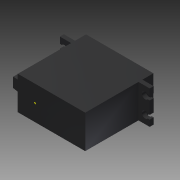
# Autodesk Inventor part: servo 13kg BMS-630MG
Saved by Autodesk Inventor 2013 (Build 170138000, 138)
## iProperties
Created: 2013-03-06
Part Number: servo 13kg BMS-630MG
Material: Generic
Document SubType Name: Modeling
Designer: Masta
Density: 1.52304 g/cm^3
Mass: 52 g
Surface Area: 75.1113 cm^2
Volume: 34.1422 cm^3
Author: Masta
Autodesk Inventor part; units mm, degrees
ref_plane "YZ Plane" through (0, 0, 0) normal (1, 0, 0) x (0, 1, 0)
ref_plane "XZ Plane" through (0, 0, 0) normal (0, 1, 0) x (-1, 0, 0)
ref_plane "XY Plane" through (0, 0, 0) normal (0, 0, 1) x (1, 0, 0)
sketch "Sketch1" plane through (0, 0, 0) normal (0, 1, 0) x (-1, 0, 0)
  line L0 (20.25, 10) -> (-20.25, 10)
  line L1 (-20.25, 10) -> (-20.25, -10)
  line L2 (-20.25, -10) -> (20.25, -10)
  line L3 (20.25, -10) -> (20.25, 10)
  line L4 (20.25, 10) -> (-20.25, -10) construction
  line L5 (-20.25, 10) -> (20.25, -10) construction
  line L6 (-27, 10) -> (-27, 6.25)
  line L7 (27, -10) -> (27, -6.25)
  line L8 (27, 10) -> (-27, -10) construction
  line L9 (-27, 10) -> (27, -10) construction
  line L10 (20.25, -10) -> (27, -10)
  line L11 (20.25, 10) -> (27, 10)
  line L12 (-20.25, 10) -> (-27, 10)
  line L13 (-20.25, -10) -> (-27, -10)
  line L14 (24.25, 5) -> (-24.25, 5) construction
  line L15 (-24.25, 5) -> (-24.25, -5) construction
  line L16 (-24.25, -5) -> (24.25, -5) construction
  line L17 (24.25, -5) -> (24.25, 5) construction
  line L18 (24.25, 5) -> (-24.25, -5) construction
  line L19 (-24.25, 5) -> (24.25, -5) construction
  circle A0 centre (-24.25, 5) radius 2
  line L20 (-27, 3.75) -> (-25.8112, 3.75)
  line L21 (-27, 6.25) -> (-25.8112, 6.25)
  line L22 (-20.25, 0) -> (20.25, 0) construction
  line L23 (0, 10) -> (0, -10) construction
  circle A1 centre (-24.25, -5) radius 2
  line L24 (-27, -3.75) -> (-25.8112, -3.75)
  line L25 (-27, -6.25) -> (-25.8112, -6.25)
  circle A2 centre (24.25, 5) radius 2
  line L26 (27, 3.75) -> (25.8112, 3.75)
  line L27 (27, 6.25) -> (25.8112, 6.25)
  line L28 (27, -6.25) -> (25.8112, -6.25)
  line L29 (27, -3.75) -> (25.8112, -3.75)
  circle A3 centre (24.25, -5) radius 2
  line L30 (-27, 3.75) -> (-27, -3.75)
  line L31 (-27, 6.25) -> (-27, 3.75)
  line L32 (-27, -6.25) -> (-27, -10)
  line L33 (-27, -3.75) -> (-27, -6.25)
  line L34 (27, -3.75) -> (27, 3.75)
  line L35 (27, -6.25) -> (27, -3.75)
  line L36 (27, 3.75) -> (27, 6.25)
  line L37 (27, 6.25) -> (27, 10)
  point P0 (0, 0)
  dimension "d0" = 40.5
  dimension "d1" = 20
  dimension "d2" = 54
  dimension "d3" = 48.5
  dimension "d4" = 10
  dimension "d12" = 2.5
  dimension "d13" = 4
  constraints: 76 end point, 32 parallel, 15 symmetric about line, 12 perpendicular, 10 midpoint, 8 point on circle, 4 centre point, 2 collinear, 2 horizontal, 1 coincident, 4 other
  measures "d0" distance of L2.end L1.end
  measures "d1" distance of L1.end L0.end
  measures "d2" distance of L7.start L8.end
  measures "d3" distance of L16.end L15.end
  measures "d4" distance of L15.end L14.end
  measures "d12" distance between parallel lines of L20 L21
  measures "d13" diameter of A0
extrude "Extrusion1" add sketch "Sketch1" along normal blind 9 and the other way blind 32 contours L3 L2 L1 L0
extrude "Extrusion2" add sketch "Sketch1" along normal blind 2.4 contours L11 L37 L27 A2 L26 L34 L29 A3 L28 L7 L10 L3 | L1 L13 L32 L25 A1 L24 L30 L20 A0 L21 L6 L12
sketch "Sketch2" plane through (0, 9, 0) normal (0, 1, 0) x (1, 0, 0)
  line L0 (-20.25, 10) -> (-20.25, -10) projected
  circle A0 centre (-9.75, 0) radius 6
  line L1 (-9.75, 0) -> (0, 0) construction
  dimension "d14" = 12
  dimension "d15" = 10.5
  constraints: 2 end point, 1 centre point, 1 perpendicular
  measures "d14" diameter of A0
  measures "d15" distance from line of L1.start L0
extrude "Extrusion3" add sketch "Sketch2" along normal blind 1.5
sketch "Sketch3" plane through (-9.75, 10.5, 0) normal (0, 1, 0) x (1, 0, 0)
  circle A0 centre (0, 0) radius 6 projected
  circle A1 centre (0, 0) radius 3
  point P0 (9.75, 0)
  dimension "d18" = 6
  constraints: 1 centre point, 1 coincident
  measures "d18" diameter of A1
extrude "Extrusion4" add sketch "Sketch3" along normal blind 4 contours A1
sketch "Sketch4" plane through (-20.25, -32, -10) normal (-1, 0, 0) x (0, 0, 1)
  line L0 (20, 32) -> (0, 32) projected
  line L1 (6.5, 3.5) -> (13.5, 3.5)
  line L2 (13.5, 3.5) -> (13.5, 8)
  line L3 (13.5, 8) -> (6.5, 8)
  line L4 (6.5, 8) -> (6.5, 3.5)
  line L5 (6.5, 3.5) -> (13.5, 8) construction
  line L6 (13.5, 3.5) -> (6.5, 8) construction
  line L7 (10, 32) -> (10, 5.75) construction
  dimension "d21" = 7
  dimension "d22" = 4.5
  dimension "d23" = 24
  constraints: 14 end point, 3 parallel, 2 midpoint, 1 horizontal, 1 perpendicular
  measures "d21" distance of L3.end L2.end
  measures "d22" distance of L2.end L1.end
  measures "d23" distance between parallel lines of L0 L3
extrude "Extrusion5" add sketch "Sketch4" along normal blind 7 draft -5
sketch "Sketch5" plane through (0, 0, 0) normal (0, 0, 1) x (1, 0, 0)
  line L0 (27, 2.4) -> (27, 0) projected
  line L1 (27, 0) -> (20.25, 0) projected
  line L2 (20.25, 0) -> (20.25, -32) projected
  line L3 (20.25, -32) -> (-20.25, -32) projected
  line L4 (-20.25, -32) -> (-20.25, -28.5) projected
  line L5 (-20.25, -28.5) -> (-27.25, -27.8876) projected
  line L6 (-27.25, -27.8876) -> (-27.25, -24.6124) projected
  line L7 (-27.25, -24.6124) -> (-20.25, -24) projected
  line L8 (-20.25, -24) -> (-20.25, 0) projected
  line L9 (-20.25, 0) -> (-27, 0) projected
  line L10 (-27, 0) -> (-27, 2.4) projected
  line L11 (-27, 2.4) -> (-20.25, 2.4) projected
  line L12 (-20.25, 2.4) -> (-20.25, 9) projected
  line L13 (-20.25, 9) -> (-15.75, 9) projected
  line L14 (-15.75, 9) -> (-15.75, 10.5) projected
  line L15 (-15.75, 10.5) -> (-12.75, 10.5) projected
  line L16 (-12.75, 10.5) -> (-12.75, 14.5) projected
  line L17 (-12.75, 14.5) -> (-6.75, 14.5) projected
  line L18 (-6.75, 14.5) -> (-6.75, 10.5) projected
  line L19 (-6.75, 10.5) -> (-3.75, 10.5) projected
  line L20 (-3.75, 10.5) -> (-3.75, 9) projected
  line L21 (-3.75, 9) -> (20.25, 9) projected
  line L22 (20.25, 9) -> (20.25, 2.4) projected
  line L23 (20.25, 2.4) -> (27, 2.4) projected
  line L24 (-27, 2.4) -> (-20.25, 3.5)
  line L25 (20.25, 3.5) -> (27, 2.4)
  point P0 (0, 0)
  dimension "d26" = 1.1
  constraints: 4 end point, 2 point on line, 1 equal length
  measures "d26" distance of L24.end L11.end
extrude "Extrusion6" add sketch "Sketch5" along normal mid plane 1.3 contours L23 L22 L25 | L24 L12 L11
sketch "Sketch6" plane through (0, 9, 0) normal (0, 1, 0) x (1, 0, 0)
  line L0 (12.3297, -9.4801) -> (12.3297, 4.6475) construction
  line L1 (12.3297, 4.6475) -> (15.9034, 4.6475) construction
  line L2 (15.9034, 4.6475) -> (15.9034, -9.4801) construction
  line L3 (15.9034, -9.4801) -> (12.3297, -9.4801) construction
  spline S0 degree 2 poles (14.1431, -7.5) (14.3325, -7.5) (14.6227, -7.6441) (14.7174, -7.7634) knots 0 0 0 1 2 2 2
  spline S1 degree 2 poles (14.7174, -7.7634) (14.8285, -7.9075) (14.9232, -8.2348) (14.9232, -8.4942) knots 0 0 0 1 2 2 2
  line L4 (14.9232, -8.4942) -> (14.9232, -9.2228)
  line L5 (14.9232, -9.2228) -> (12.3832, -9.2228)
  line L6 (12.3832, -9.2228) -> (12.3832, -8.5497)
  spline S2 degree 2 poles (12.3832, -8.5497) (12.3832, -8.278) (12.4182, -8.0063) (12.4861, -7.8828) knots 0 0 0 1 2 2 2
  spline S3 degree 2 poles (12.4861, -7.8828) (12.5582, -7.7449) (12.7949, -7.6194) (12.9554, -7.6194) knots 0 0 0 1 2 2 2
  spline S4 degree 2 poles (12.9554, -7.6194) (13.1345, -7.6194) (13.4185, -7.8087) (13.4988, -7.9755) knots 0 0 0 1 2 2 2
  line L7 (13.4988, -7.9755) -> (13.5112, -7.9755)
  spline S5 degree 2 poles (13.5112, -7.9755) (13.5729, -7.749) (13.9002, -7.5) (14.1431, -7.5) knots 0 0 0 1 2 2 2
  spline S6 degree 2 poles (14.1575, -7.852) (14.0134, -7.852) (13.8282, -7.9343) (13.7623, -8.0578) knots 0 0 0 1 2 2 2
  spline S7 degree 2 poles (13.7623, -8.0578) (13.7211, -8.1381) (13.6964, -8.3274) (13.6964, -8.5024) knots 0 0 0 1 2 2 2
  line L8 (13.6964, -8.5024) -> (13.6964, -8.8852)
  line L9 (13.6964, -8.8852) -> (14.635, -8.8852)
  line L10 (14.635, -8.8852) -> (14.635, -8.6115)
  spline S8 degree 2 poles (14.635, -8.6115) (14.635, -8.3892) (14.5939, -8.1339) (14.528, -8.0351) knots 0 0 0 1 2 2 2
  spline S9 degree 2 poles (14.528, -8.0351) (14.4601, -7.9405) (14.2913, -7.852) (14.1575, -7.852) knots 0 0 0 1 2 2 2
  spline S10 degree 2 poles (13.0028, -7.9713) (12.9122, -7.9713) (12.7763, -8.0331) (12.7372, -8.101) knots 0 0 0 1 2 2 2
  spline S11 degree 2 poles (12.7372, -8.101) (12.692, -8.1833) (12.6714, -8.383) (12.6714, -8.5621) knots 0 0 0 1 2 2 2
  line L11 (12.6714, -8.5621) -> (12.6714, -8.8852)
  line L12 (12.6714, -8.8852) -> (13.4144, -8.8852)
  line L13 (13.4144, -8.8852) -> (13.4144, -8.5024)
  spline S12 degree 2 poles (13.4144, -8.5024) (13.4144, -8.3439) (13.3815, -8.1936) (13.33, -8.1134) knots 0 0 0 1 2 2 2
  spline S13 degree 2 poles (13.33, -8.1134) (13.2806, -8.0351) (13.1221, -7.9713) (13.0028, -7.9713) knots 0 0 0 1 2 2 2
  line L14 (14.9232, -4.9867) -> (14.9232, -5.3243)
  line L15 (14.9232, -5.3243) -> (12.7352, -5.3243)
  line L16 (12.7352, -5.3243) -> (14.2234, -5.9871)
  line L17 (14.2234, -5.9871) -> (14.2234, -6.1929)
  line L18 (14.2234, -6.1929) -> (12.7352, -6.8495)
  line L19 (12.7352, -6.8495) -> (14.9232, -6.8495)
  line L20 (14.9232, -6.8495) -> (14.9232, -7.1645)
  line L21 (14.9232, -7.1645) -> (12.3832, -7.1645)
  line L22 (12.3832, -7.1645) -> (12.3832, -6.7034)
  line L23 (12.3832, -6.7034) -> (13.7973, -6.0694)
  line L24 (13.7973, -6.0694) -> (12.3832, -5.456)
  line L25 (12.3832, -5.456) -> (12.3832, -4.9867)
  line L26 (12.3832, -4.9867) -> (14.9232, -4.9867)
  spline S14 degree 2 poles (14.9685, -3.7641) (14.9685, -4.0399) (14.8532, -4.4269) (14.7709, -4.5977) knots 0 0 0 1 2 2 2
  line L27 (14.7709, -4.5977) -> (14.3469, -4.5977)
  line L28 (14.3469, -4.5977) -> (14.3469, -4.573)
  spline S15 degree 2 poles (14.3469, -4.573) (14.5033, -4.4063) (14.6762, -3.9843) (14.6762, -3.7888) knots 0 0 0 1 2 2 2
  spline S16 degree 2 poles (14.6762, -3.7888) (14.6762, -3.5088) (14.4436, -3.2227) (14.2522, -3.2227) knots 0 0 0 1 2 2 2
  spline S17 degree 2 poles (14.2522, -3.2227) (14.0999, -3.2227) (13.9105, -3.373) (13.8632, -3.5356) knots 0 0 0 1 2 2 2
  spline S18 degree 2 poles (13.8632, -3.5356) (13.8302, -3.6529) (13.7849, -3.8485) (13.7479, -3.9946) knots 0 0 0 1 2 2 2
  spline S19 degree 2 poles (13.7479, -3.9946) (13.7129, -4.1263) (13.6079, -4.3342) (13.5235, -4.4145) knots 0 0 0 1 2 2 2
  spline S20 degree 2 poles (13.5235, -4.4145) (13.4391, -4.4927) (13.2127, -4.5792) (13.0645, -4.5792) knots 0 0 0 1 2 2 2
  spline S21 degree 2 poles (13.0645, -4.5792) (12.7558, -4.5792) (12.3379, -4.0975) (12.3379, -3.725) knots 0 0 0 1 2 2 2
  spline S22 degree 2 poles (12.3379, -3.725) (12.3379, -3.5109) (12.4223, -3.1322) (12.5026, -2.9696) knots 0 0 0 1 2 2 2
  line L29 (12.5026, -2.9696) -> (12.906, -2.9696)
  line L30 (12.906, -2.9696) -> (12.906, -2.9943)
  spline S23 degree 2 poles (12.906, -2.9943) (12.7949, -3.1157) (12.6302, -3.4944) (12.6302, -3.7023) knots 0 0 0 1 2 2 2
  spline S24 degree 2 poles (12.6302, -3.7023) (12.6302, -3.937) (12.8504, -4.2272) (13.0295, -4.2272) knots 0 0 0 1 2 2 2
  spline S25 degree 2 poles (13.0295, -4.2272) (13.1901, -4.2272) (13.3815, -4.0564) (13.4247, -3.8958) knots 0 0 0 1 2 2 2
  spline S26 degree 2 poles (13.4247, -3.8958) (13.4535, -3.7888) (13.5276, -3.478) (13.5585, -3.375) knots 0 0 0 1 2 2 2
  spline S27 degree 2 poles (13.5585, -3.375) (13.6388, -3.1136) (13.962, -2.8708) (14.1987, -2.8708) knots 0 0 0 1 2 2 2
  spline S28 degree 2 poles (14.1987, -2.8708) (14.3489, -2.8708) (14.6371, -2.9922) (14.7379, -3.1013) knots 0 0 0 1 2 2 2
  spline S29 degree 2 poles (14.7379, -3.1013) (14.8491, -3.2227) (14.9685, -3.5315) (14.9685, -3.7641) knots 0 0 0 1 2 2 2
  line L31 (13.9661, -1.6687) -> (13.9661, -2.6299)
  line L32 (13.9661, -2.6299) -> (13.6573, -2.6299)
  line L33 (13.6573, -2.6299) -> (13.6573, -1.6687)
  line L34 (13.6573, -1.6687) -> (13.9661, -1.6687)
  spline S30 degree 2 poles (14.0999, 0.2744) (14.2954, 0.2744) (14.6268, 0.1447) (14.7379, 0.0356) knots 0 0 0 1 2 2 2
  spline S31 degree 2 poles (14.7379, 0.0356) (14.8553, -0.0776) (14.9767, -0.3616) (14.9767, -0.5325) knots 0 0 0 1 2 2 2
  spline S32 degree 2 poles (14.9767, -0.5325) (14.9767, -0.7033) (14.8614, -0.9853) (14.7462, -1.0923) knots 0 0 0 1 2 2 2
  spline S33 degree 2 poles (14.7462, -1.0923) (14.6083, -1.2241) (14.1451, -1.3723) (13.8076, -1.3723) knots 0 0 0 1 2 2 2
  spline S34 degree 2 poles (13.8076, -1.3723) (13.4762, -1.3723) (12.9431, -1.2364) (12.7455, -1.0944) knots 0 0 0 1 2 2 2
  spline S35 degree 2 poles (12.7455, -1.0944) (12.552, -0.9565) (12.3359, -0.5201) (12.3359, -0.234) knots 0 0 0 1 2 2 2
  spline S36 degree 2 poles (12.3359, -0.234) (12.3359, -0.1496) (12.3523, -0.0014) (12.3708, 0.0542) knots 0 0 0 1 2 2 2
  line L35 (12.3708, 0.0542) -> (12.6981, 0.0542)
  line L36 (12.6981, 0.0542) -> (12.6981, 0.0397)
  spline S37 degree 2 poles (12.6981, 0.0397) (12.6734, -0.0076) (12.6302, -0.1805) (12.6302, -0.2793) knots 0 0 0 1 2 2 2
  spline S38 degree 2 poles (12.6302, -0.2793) (12.6302, -0.5963) (13.0583, -0.9853) (13.4782, -1.0224) knots 0 0 0 1 2 2 2
  spline S39 degree 2 poles (13.4782, -1.0224) (13.3938, -0.9009) (13.3012, -0.6457) (13.3012, -0.4934) knots 0 0 0 1 2 2 2
  spline S40 degree 2 poles (13.3012, -0.4934) (13.3012, -0.3452) (13.3609, -0.1229) (13.4515, -0.0014) knots 0 0 0 1 2 2 2
  spline S41 degree 2 poles (13.4515, -0.0014) (13.5565, 0.1385) (13.8817, 0.2744) (14.0999, 0.2744) knots 0 0 0 1 2 2 2
  spline S42 degree 2 poles (14.1143, -0.0714) (13.9578, -0.0714) (13.7458, -0.1537) (13.6717, -0.2443) knots 0 0 0 1 2 2 2
  spline S43 degree 2 poles (13.6717, -0.2443) (13.6182, -0.3122) (13.5832, -0.481) (13.5832, -0.5695) knots 0 0 0 1 2 2 2
  spline S44 degree 2 poles (13.5832, -0.5695) (13.5832, -0.6889) (13.6553, -0.9133) (13.7232, -1.0224) knots 0 0 0 1 2 2 2
  spline S45 degree 2 poles (13.7232, -1.0224) (13.7602, -1.0244) (13.8302, -1.0285) (13.8837, -1.0285) knots 0 0 0 1 2 2 2
  spline S46 degree 2 poles (13.8837, -1.0285) (14.1472, -1.0285) (14.4704, -0.9256) (14.5548, -0.8474) knots 0 0 0 1 2 2 2
  spline S47 degree 2 poles (14.5548, -0.8474) (14.635, -0.7754) (14.6988, -0.6189) (14.6988, -0.5304) knots 0 0 0 1 2 2 2
  spline S48 degree 2 poles (14.6988, -0.5304) (14.6988, -0.3246) (14.4066, -0.0714) (14.1143, -0.0714) knots 0 0 0 1 2 2 2
  spline S49 degree 2 poles (12.624, 1.2603) (12.624, 1.1677) (12.6693, 0.9845) (12.7043, 0.896) knots 0 0 0 1 2 2 2
  spline S50 degree 2 poles (12.7043, 0.896) (12.7393, 0.8137) (12.8134, 0.6922) (12.8463, 0.6449) knots 0 0 0 1 2 2 2
  line L37 (12.8463, 0.6449) -> (12.8463, 0.6243)
  line L38 (12.8463, 0.6243) -> (12.4861, 0.6243)
  spline S51 degree 2 poles (12.4861, 0.6243) (12.4264, 0.7355) (12.3297, 1.1163) (12.3297, 1.2871) knots 0 0 0 1 2 2 2
  spline S52 degree 2 poles (12.3297, 1.2871) (12.3297, 1.46) (12.3997, 1.7173) (12.4738, 1.8223) knots 0 0 0 1 2 2 2
  spline S53 degree 2 poles (12.4738, 1.8223) (12.554, 1.9334) (12.7866, 2.0487) (12.9431, 2.0487) knots 0 0 0 1 2 2 2
  spline S54 degree 2 poles (12.9431, 2.0487) (13.153, 2.0487) (13.47, 1.7729) (13.5112, 1.5794) knots 0 0 0 1 2 2 2
  line L39 (13.5112, 1.5794) -> (13.5359, 1.5794)
  spline S55 degree 2 poles (13.5359, 1.5794) (13.5523, 1.6597) (13.6264, 1.8429) (13.7005, 1.9211) knots 0 0 0 1 2 2 2
  spline S56 degree 2 poles (13.7005, 1.9211) (13.7726, 1.9993) (14.0031, 2.0981) (14.1698, 2.0981) knots 0 0 0 1 2 2 2
  spline S57 degree 2 poles (14.1698, 2.0981) (14.3407, 2.0981) (14.6309, 1.9808) (14.7421, 1.8737) knots 0 0 0 1 2 2 2
  spline S58 degree 2 poles (14.7421, 1.8737) (14.8573, 1.7626) (14.9767, 1.4477) (14.9767, 1.248) knots 0 0 0 1 2 2 2
  spline S59 degree 2 poles (14.9767, 1.248) (14.9767, 1.0566) (14.8841, 0.682) (14.8203, 0.5543) knots 0 0 0 1 2 2 2
  line L40 (14.8203, 0.5543) -> (14.4601, 0.5543)
  line L41 (14.4601, 0.5543) -> (14.4601, 0.579)
  spline S60 degree 2 poles (14.4601, 0.579) (14.5383, 0.6861) (14.6824, 1.0483) (14.6824, 1.2274) knots 0 0 0 1 2 2 2
  spline S61 degree 2 poles (14.6824, 1.2274) (14.6824, 1.3324) (14.6165, 1.5423) (14.5403, 1.6123) knots 0 0 0 1 2 2 2
  spline S62 degree 2 poles (14.5403, 1.6123) (14.4642, 1.6803) (14.2831, 1.7523) (14.1451, 1.7523) knots 0 0 0 1 2 2 2
  spline S63 degree 2 poles (14.1451, 1.7523) (14.0072, 1.7523) (13.8282, 1.672) (13.7767, 1.6) knots 0 0 0 1 2 2 2
  spline S64 degree 2 poles (13.7767, 1.6) (13.7252, 1.5279) (13.6861, 1.3324) (13.6861, 1.2171) knots 0 0 0 1 2 2 2
  line L42 (13.6861, 1.2171) -> (13.6861, 1.073)
  line L43 (13.6861, 1.073) -> (13.4041, 1.073)
  line L44 (13.4041, 1.073) -> (13.4041, 1.1862)
  spline S65 degree 2 poles (13.4041, 1.1862) (13.4041, 1.4147) (13.186, 1.7029) (12.9781, 1.7029) knots 0 0 0 1 2 2 2
  spline S66 degree 2 poles (12.9781, 1.7029) (12.8813, 1.7029) (12.7434, 1.6288) (12.7022, 1.5691) knots 0 0 0 1 2 2 2
  spline S67 degree 2 poles (12.7022, 1.5691) (12.659, 1.5053) (12.624, 1.3489) (12.624, 1.2603) knots 0 0 0 1 2 2 2
  spline S68 degree 2 poles (13.6532, 4.0618) (14.3366, 4.0618) (14.9767, 3.6645) (14.9767, 3.2508) knots 0 0 0 1 2 2 2
  spline S69 degree 2 poles (14.9767, 3.2508) (14.9767, 2.8309) (14.3242, 2.4377) (13.6553, 2.4377) knots 0 0 0 1 2 2 2
  spline S70 degree 2 poles (13.6553, 2.4377) (12.9678, 2.4377) (12.3317, 2.835) (12.3317, 3.2508) knots 0 0 0 1 2 2 2
  spline S71 degree 2 poles (12.3317, 3.2508) (12.3317, 3.6686) (12.9904, 4.0618) (13.6532, 4.0618) knots 0 0 0 1 2 2 2
  spline S72 degree 2 poles (14.4271, 3.6254) (14.3016, 3.6748) (13.9146, 3.716) (13.6532, 3.716) knots 0 0 0 1 2 2 2
  spline S73 degree 2 poles (13.6532, 3.716) (13.3918, 3.716) (13.0069, 3.6748) (12.8772, 3.6233) knots 0 0 0 1 2 2 2
  spline S74 degree 2 poles (12.8772, 3.6233) (12.7475, 3.5719) (12.6137, 3.3928) (12.6137, 3.2508) knots 0 0 0 1 2 2 2
  spline S75 degree 2 poles (12.6137, 3.2508) (12.6137, 3.1087) (12.7475, 2.9256) (12.8813, 2.872) knots 0 0 0 1 2 2 2
  spline S76 degree 2 poles (12.8813, 2.872) (13.011, 2.8206) (13.4062, 2.7835) (13.6553, 2.7835) knots 0 0 0 1 2 2 2
  spline S77 degree 2 poles (13.6553, 2.7835) (13.9228, 2.7835) (14.281, 2.8165) (14.421, 2.87) knots 0 0 0 1 2 2 2
  spline S78 degree 2 poles (14.421, 2.87) (14.5527, 2.9194) (14.6947, 3.1026) (14.6947, 3.2508) knots 0 0 0 1 2 2 2
  spline S79 degree 2 poles (14.6947, 3.2508) (14.6947, 3.3907) (14.5609, 3.5739) (14.4271, 3.6254) knots 0 0 0 1 2 2 2
  line L45 (14.9232, 6.6368) -> (14.9232, 6.2992)
  line L46 (14.9232, 6.2992) -> (12.7352, 6.2992)
  line L47 (12.7352, 6.2992) -> (14.2234, 5.6364)
  line L48 (14.2234, 5.6364) -> (14.2234, 5.4306)
  line L49 (14.2234, 5.4306) -> (12.7352, 4.7739)
  line L50 (12.7352, 4.7739) -> (14.9232, 4.7739)
  line L51 (14.9232, 4.7739) -> (14.9232, 4.459)
  line L52 (14.9232, 4.459) -> (12.3832, 4.459)
  line L53 (12.3832, 4.459) -> (12.3832, 4.9201)
  line L54 (12.3832, 4.9201) -> (13.7973, 5.5541)
  line L55 (13.7973, 5.5541) -> (12.3832, 6.1674)
  line L56 (12.3832, 6.1674) -> (12.3832, 6.6368)
  line L57 (12.3832, 6.6368) -> (14.9232, 6.6368)
  spline S80 degree 2 poles (14.9726, 8.2155) (14.9726, 7.9459) (14.8079, 7.4992) (14.6412, 7.3386) knots 0 0 0 1 2 2 2
  spline S81 degree 2 poles (14.6412, 7.3386) (14.4724, 7.1781) (13.9743, 7.0073) (13.6511, 7.0073) knots 0 0 0 1 2 2 2
  spline S82 degree 2 poles (13.6511, 7.0073) (13.3444, 7.0073) (12.8587, 7.1802) (12.6858, 7.3407) knots 0 0 0 1 2 2 2
  spline S83 degree 2 poles (12.6858, 7.3407) (12.5191, 7.4951) (12.3379, 7.9479) (12.3379, 8.2176) knots 0 0 0 1 2 2 2
  spline S84 degree 2 poles (12.3379, 8.2176) (12.3379, 8.3472) (12.375, 8.5819) (12.4079, 8.6889) knots 0 0 0 1 2 2 2
  spline S85 degree 2 poles (12.4079, 8.6889) (12.4326, 8.7754) (12.5232, 8.9853) (12.5561, 9.0491) knots 0 0 0 1 2 2 2
  line L58 (12.5561, 9.0491) -> (12.9637, 9.0491)
  line L59 (12.9637, 9.0491) -> (12.9637, 9.0203)
  spline S86 degree 2 poles (12.9637, 9.0203) (12.9081, 8.9565) (12.8072, 8.8227) (12.7496, 8.6992) knots 0 0 0 1 2 2 2
  spline S87 degree 2 poles (12.7496, 8.6992) (12.6981, 8.5963) (12.6302, 8.3308) (12.6302, 8.1785) knots 0 0 0 1 2 2 2
  spline S88 degree 2 poles (12.6302, 8.1785) (12.6302, 7.8121) (13.1818, 7.3592) (13.6408, 7.3592) knots 0 0 0 1 2 2 2
  spline S89 degree 2 poles (13.6408, 7.3592) (13.8961, 7.3592) (14.2789, 7.4786) (14.4107, 7.5918) knots 0 0 0 1 2 2 2
  spline S90 degree 2 poles (14.4107, 7.5918) (14.5424, 7.7009) (14.6803, 8.0097) (14.6803, 8.2032) knots 0 0 0 1 2 2 2
  spline S91 degree 2 poles (14.6803, 8.2032) (14.6803, 8.3452) (14.6391, 8.6292) (14.598, 8.726) knots 0 0 0 1 2 2 2
  line L60 (14.598, 8.726) -> (13.9414, 8.726)
  line L61 (13.9414, 8.726) -> (13.9414, 8.1373)
  line L62 (13.9414, 8.1373) -> (13.645, 8.1373)
  line L63 (13.645, 8.1373) -> (13.645, 9.0594)
  line L64 (13.645, 9.0594) -> (14.7544, 9.0594)
  spline S92 degree 2 poles (14.7544, 9.0594) (14.7832, 8.9956) (14.8717, 8.7774) (14.8985, 8.6848) knots 0 0 0 1 2 2 2
  spline S93 degree 2 poles (14.8985, 8.6848) (14.9355, 8.5592) (14.9726, 8.3575) (14.9726, 8.2155) knots 0 0 0 1 2 2 2
  point P0 (0, 0)
  constraints: 2 other
emboss "Emboss1" sketch "Sketch6" operation cut depth 0.1 direction (0, -1, 0)
hole "Hole1" at (-9.75, 14.5, 0) direction (0, -1, 0) diameter 2.459 depth 8 tip angle 118 thread size "M3x0.5" class "6H" standard "ISO Metric profile"
sketch "Sketch7" plane through (0, -32, 0) normal (0, -1, 0) x (1, 0, 0)
  line L0 (20.25, 10) -> (-20.25, 10) projected
  line L1 (-20.25, 10) -> (-20.25, -10) projected
  line L2 (-20.25, -10) -> (20.25, -10) projected
  line L3 (20.25, -10) -> (20.25, 10) projected
  point P0 (0, 0)
  point P1 (-9.75, 0)
body "Solid1"
